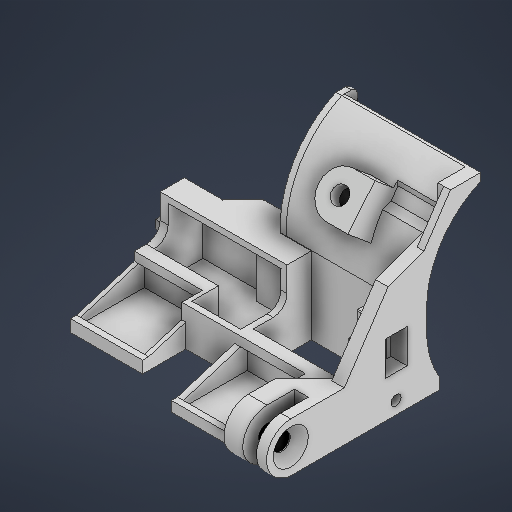
# Autodesk Inventor part: body-main2
Saved by Autodesk Inventor 2025 (Build 290162000, 162)
## iProperties
Created: 2025-03-21
Part Number: body-main2
Material: Všeobecné
Document SubType Name: Modeling
Designer: Simak
Density: 1 g/cm^3
Appearance: Výchozí
Author: Simak
Autodesk Inventor part; units mm, degrees
ref_plane "YZ Plane" through (0, 0, 0) normal (1, 0, 0) x (0, 1, 0)
ref_plane "XZ Plane" through (0, 0, 0) normal (0, 1, 0) x (-1, 0, 0)
ref_plane "XY Plane" through (0, 0, 0) normal (0, 0, 1) x (1, 0, 0)
sketch "Náčrt1" plane through (0, 0, 0) normal (1, 0, 0) x (0, 1, 0)
  circle A0 centre (13.5, 0) radius 16.5 construction
  circle A1 centre (15.5, 0) radius 16.5 construction
  circle A2 centre (11.5, 0) radius 16.5 construction
  line L0 (15.5, 16.5) -> (11.5, 16.5) construction
  line L1 (15.5, -16.5) -> (11.5, -16.5) construction
  circle A3 centre (5, 45.139) radius 5
  line L2 (0, 0) -> (0, 45.139)
  line L3 (10, 34.353) -> (22.965058, 25.70965)
  line L4 (10, 34.353) -> (10, 45.139)
  line L5 (22.965058, 25.70965) -> (27.5, 13.25)
  line L6 (27.5, 13.25) -> (33.5, 13.25)
  line L7 (33.5, 13.25) -> (25.577679, 18.531534)
  line L8 (33.5, 13.25) -> (33.5, 7.193747)
  line L9 (29, 13.25) -> (27.01942, 14.570383)
  arc A4 (13.5, -17.888544) -> (15.5, 18) centre (15.5, 0) ccw
  arc A5 (11.5, 18) -> (13.5, -17.888544) centre (11.5, 0) ccw
  line L10 (15.5, 18) -> (11.5, 18)
  line L11 (2.348497, 15.5) -> (0, 15.5)
  line L12 (33.5, 7.193747) -> (32, 7.193747)
  arc A6 (13.5, -19.497692) -> (15.5, 19.6) centre (15.5, 0) ccw
  arc A7 (11.5, 19.6) -> (13.5, -19.497692) centre (11.5, 0) ccw
  line L13 (11.5, 19.6) -> (15.5, 19.6)
  line L14 (21.6, 28.6) -> (0, 28.6) construction
  line L15 (0, 28.6) -> (0, 19.6)
  line L16 (0, 19.6) -> (21.6, 19.6)
  line L17 (21.6, 19.6) -> (21.6, 28.6) construction
  line L18 (35.6, 21.5) -> (34, 21.5) construction
  line L19 (34, 21.5) -> (34, -16) construction
  line L20 (34, -16) -> (35.6, -16) construction
  line L21 (35.6, -16) -> (35.6, 21.5) construction
  line L22 (35.6, 17.75) -> (34, 17.75) construction
  line L23 (33.21956, 14.55) -> (26.524235, 14.55) construction
  line L24 (10, 39.639) -> (0, 39.639)
  line L25 (10, 34.353) -> (9.85, 34.453)
  line L26 (9.85, 34.453) -> (9.85, 39.639)
  point P0 (26.391657, 16.295147)
  point P1 (33.5, 7.756288)
  point P2 (29.942905, 13.25)
  dimension "d0" = 33
  dimension "d1" = 2
  dimension "d2" = 2
  dimension "d3" = 13.5
  dimension "d4" = 10
  dimension "d5" = 45.139
  dimension "d6" = 10.786
  dimension "d8" = 123.69
  dimension "d10" = 13.25
  dimension "d11" = 33.5
  dimension "d12" = 6
  dimension "d16" = 1.5
  dimension "d17" = 36
  dimension "d18" = 36
  dimension "d20" = 1.5
  dimension "d21" = 1.6
  dimension "d23" = 9
  dimension "d24" = 21.6
  dimension "d25" = 0.5
  dimension "d26" = 1.6
  dimension "d27" = 37.5
  dimension "d28" = 3.75
  dimension "d29" = 20.5
  dimension "d30" = 3.2
  dimension "d41" = 5.5
  dimension "d45" = 9.85
  dimension "d86" = 70
  dimension "d103" = 15.5
  constraints: 54 end point, 17 point on circle, 11 point on line, 8 centre point, 8 perpendicular, 7 horizontal, 5 parallel, 5 tangent, 3 horizontal alignment, 3 vertical, 2 coincident, 2 collinear, 2 equal radius, 2 other
  measures "d0" diameter of A0
  measures "d1" distance of A0.centre A1.centre
  measures "d2" distance of A0.centre A2.centre
  measures "d3" distance of A0.centre L2.start
  measures "d4" diameter of A3
  measures "d5" vertical distance of A3.centre A0.centre
  measures "d6" vertical distance of A3.centre L3.start
  measures "d8" angle of L4 L3
  measures "d10" distance from line of A1.centre L6
  measures "d11" distance from line of L2 L6.end
  measures "d12" distance of L5.end L6.end
  measures "d16" distance of L5.end L9.start
  measures "d17" diameter of A4
  measures "d18" diameter of A5
  measures "d20" distance of L8.end L12.end
  measures "d21" radial gap between concentric circles of A4 A6
  measures "d23" distance of L16.end L14.start
  measures "d24" distance of L14.start L14.end
  measures "d25" distance between parallel lines of L20 L1
  measures "d26" distance of L19.end L20.end
  measures "d27" distance of L20.end L18.start
  measures "d28" distance between parallel lines of L18 L22
  measures "d29" distance from line of L19 A0.centre
  measures "d30" distance between parallel lines of L22 L23
  measures "d41" distance from line of A3.centre L24
  measures "d45" distance between parallel lines of L2 L26
  measures "d86" angle of L6 L5
  measures "d103" distance from line of A0.centre L11
extrude "Vysunutí1" add sketch "Náčrt1" against normal blind 2.5 contours L24 L26 L25 L3 L5 A6 L13 L16 L2 | L16 A7 L2 | A7 L13 A6 L5 A4 L10 A5 L11 L2 | L8 A6 L6 | L9 L6 A4 L5 | A6 L8 L12 A4 L6
extrude "Vysunutí3" add sketch "Náčrt1" against normal blind 49.5 contours L16 A7 L2 | A7 L13 A6 L5 A4 L10 A5 L11 L2 | A6 L6 L9 L5 | L9 L6 A4 L5 | A6 L8 L12 A4 L6
extrude "Vysunutí4" cut sketch "Náčrt1" against normal blind 10.5 contours A6 L6 L9 L5
extrude "Vysunutí5" add sketch "Náčrt1" against normal blind 1.35 contours L7 L6 A6 L5 | A6 L6 L9 L5
sketch "Náčrt2" plane through (0, 0, 0) normal (1, 0, 0) x (0, 0, -1)
  circle A0 centre (-45.139, 5) radius 4.85
  line L0 (-46.797798, 0.442491) -> (-45.582064, 0)
  line L1 (-19.6, 0) -> (-39.639, 0)
  line L2 (-39.639, 0) -> (-45.582064, 0)
  line L3 (-39.639, 9.85) -> (-39.639, 0)
  line L4 (-39.639, 9.85) -> (-45.139, 9.85)
  line L5 (-45.139, 8.889087) -> (-49.028087, 5)
  line L6 (-49.028087, 5) -> (-45.139, 1.110913)
  line L7 (-45.139, 1.110913) -> (-41.249913, 5)
  line L8 (-41.249913, 5) -> (-45.139, 8.889087)
  line L9 (-45.139, 8.889087) -> (-45.139, 5) construction
  line L10 (-45.139, 5) -> (-41.249913, 5) construction
  line L11 (-45.139, 5) -> (-45.139, 1.110913) construction
  point P0 (0, 0)
  dimension "d42" = 9.7
  dimension "d44" = 20
  dimension "d47" = 5.5
  constraints: 20 end point, 5 equal length, 4 perpendicular, 2 point on circle, 2 tangent, 1 centre point, 1 coincident, 1 collinear, 1 vertical
  measures "d42" diameter of A0
  measures "d44" angle of L2 L0
  measures "d47" distance of L7.end L5.start
extrude "Vysunutí6" add sketch "Náčrt2" against normal blind 8.5 contours A0 | A0 L4 L3 L2 L0 | L8 L7 L6 L5
sketch "Náčrt3" plane through (0, 0, 0) normal (1, 0, 0) x (0, 0, -1)
  arc A0 (-45.139, 9.85) -> (-46.797798, 0.442491) centre (-45.139, 5) ccw construction
  point P0 (0, 0)
  constraints: 1 coincident
hole "Díra1" at (0, 5, 45.139) direction (-1, 0, 0) diameter 3.4 end through all countersink diameter 7 countersink angle 90
sketch "Náčrt4" plane through (-8.5, 0, 0) normal (-1, 0, 0) x (0, 0, 1)
  line L0 (45.139, 1.110913) -> (41.249913, 5)
  line L1 (41.249913, 5) -> (45.139, 8.889087)
  line L2 (45.139, 8.889087) -> (49.028087, 5)
  line L3 (49.028087, 5) -> (45.139, 1.110913)
  point P0 (0, 0)
extrude "Vysunutí7" cut sketch "Náčrt4" against normal blind 2
sketch "Náčrt5" plane through (-2.5, 9.85, 34.453) normal (0, 1, 0) x (1, 0, 0)
  line L0 (2.5, -15.536) -> (-6, -15.536)
  line L1 (0.5, -15.536) -> (0.5, -5.186)
  line L2 (0.7, -12.386) -> (0.7, -8.986)
  line L3 (0.5, -5.186) -> (-2.25, -5.186)
  line L4 (-2.25, -5.186) -> (-2.25, -15.536)
  line L5 (2.5, 0) -> (2.5, -10.686)
  line L6 (2.5, -10.686) -> (-6, -10.686)
  line L7 (-6, -10.686) -> (-6, -5.186)
  line L8 (-6, -5.186) -> (0, 0.814)
  line L9 (0, 0) -> (0, 8.74335)
  line L10 (0, -5.186) -> (-6, -5.186)
  line L11 (0, -5.186) -> (0, 0)
  point P0 (2.5, 34.453)
  dimension "d59" = 2
  dimension "d60" = 2.75
  dimension "d61" = 5.5
  dimension "d62" = 45
  constraints: 8 end point, 2 perpendicular, 2 point on line, 1 parallel
  measures "d59" distance between parallel lines of L5 L1
  measures "d60" distance of L1.end L3.end
  measures "d61" distance between parallel lines of L3 L6
  measures "d62" angle of L10 L8
extrude "Vysunutí8" add sketch "Náčrt5" against normal up to surface (9.85 mm away) contours L10 L8 L9 L11 L3
extrude "Vysunutí9" cut sketch "Náčrt5" against normal through all contours L0 L4 L6 L1 | L6 L4 L3 L1
sketch "Náčrt6" plane through (-2.5, 0, 0) normal (-1, 0, 0) x (0, 0, 1)
  line L0 (19.6, 21.6) -> (28.6, 21.6)
  line L1 (28.6, 21.6) -> (28.6, 0)
  line L2 (19.6, 0) -> (19.6, 21.6)
  line L3 (19.6, 0) -> (33.639, 0)
  circle A0 centre (24.1, 2.54) radius 1
  line L4 (22.9, 13.2) -> (25.3, 13.2)
  line L5 (25.3, 13.2) -> (25.3, 8.4)
  line L6 (25.3, 8.4) -> (22.9, 8.4)
  line L7 (22.9, 8.4) -> (22.9, 13.2)
  line L8 (21.9, 14.2) -> (26.3, 14.2)
  line L9 (26.3, 14.2) -> (26.3, 7.4)
  line L10 (26.3, 7.4) -> (21.9, 7.4)
  line L11 (21.9, 7.4) -> (21.9, 14.2)
  line L12 (34.453, 9.85) -> (25.70965, 22.965058)
  line L13 (19.6, 18.85) -> (28.6, 18.85)
  arc A1 (13.25, 29.942905) -> (7.756288, 33.5) centre (0, 15.5) ccw
  arc A2 (19.6, 15.5) -> (7.756288, 33.5) centre (0, 15.5) ccw
  arc A3 (19.6, 15.5) -> (16.295147, 26.391657) centre (0, 15.5) ccw
  arc A4 (16.295147, 26.391657) -> (13.25, 29.942905) centre (0, 15.5) ccw
  line L14 (19.6, 18.85) -> (19.31159, 18.85)
  point P0 (0, 0)
  point P1 (24.1, 21.6)
  point P2 (24.1, 13.2)
  point P3 (28.453015, 18.85)
  point P4 (28.6, 18.629522)
  dimension "d67" = 2.54
  dimension "d68" = 2
  dimension "d69" = 2.4
  dimension "d70" = 4.8
  dimension "d71" = 8.4
  dimension "d72" = 1
  dimension "d77" = 2.75
  constraints: 20 end point, 4 parallel, 3 horizontal, 2 midpoint, 2 perpendicular, 2 point on line, 2 vertical alignment, 1 centre point, 1 point on circle, 3 other
  measures "d67" distance from line of L3 A0.centre
  measures "d68" diameter of A0
  measures "d69" distance of L4.start L4.end
  measures "d70" distance of L4.end L5.end
  measures "d71" distance between parallel lines of L3 L6
  measures "d72" distance between parallel lines of L7 L11
  measures "d77" distance between parallel lines of L0 L13
extrude "Vysunutí10" add sketch "Náčrt6" along normal blind 2.5 contours L13 L12 L1 L3 L2 | L2 A2 L14
extrude "Vysunutí11" cut sketch "Náčrt6" against normal through all contours A0 | L4 L5 L6 L7 | L8 L9 L10 L11
sketch "Náčrt7" plane through (-5, 0, 0) normal (-1, 0, 0) x (0, 0, 1)
  line L0 (19.6, 0) -> (19.6, 15.5)
  line L1 (19.6, 3.25) -> (28.6, 3.25)
  line L2 (28.6, 0) -> (28.6, 18.629522)
  line L3 (28.6, 5.5) -> (27.1, 5.5)
  line L4 (27.1, 5.5) -> (27.1, 13)
  line L5 (27.1, 13) -> (28.6, 13)
  line L6 (19.6, 13) -> (21.1, 13)
  line L7 (21.1, 13) -> (21.1, 5.5)
  line L8 (21.1, 5.5) -> (19.6, 5.5)
  circle A0 centre (24.1, 2.54) radius 1
  line L9 (19.6, 0) -> (28.6, 0)
  circle A1 centre (24.1, 2.54) radius 2
  line L10 (19.6, 0) -> (19.6, 15.5)
  line L11 (19.6, 0) -> (28.6, 0)
  line L12 (28.6, 0) -> (28.6, 18.629522)
  line L13 (28.453015, 18.85) -> (19.31159, 18.85)
  line L14 (21.9, 14.2) -> (26.3, 14.2)
  line L15 (26.3, 14.2) -> (26.3, 7.4)
  line L16 (26.3, 7.4) -> (21.9, 7.4)
  line L17 (21.9, 7.4) -> (21.9, 14.2)
  circle A2 centre (24.1, 2.54) radius 1
  line L18 (28.6, 18.629522) -> (28.453015, 18.85)
  arc A3 (19.6, 15.5) -> (19.31159, 18.85) centre (0, 15.5) ccw
  point P0 (0, 0)
  point P1 (28.6, 18.85)
  point P2 (28.6, 18.85)
  point P3 (22.230267, 3.25)
  point P4 (25.969733, 3.25)
  dimension "d78" = 1.5
  dimension "d79" = 7.5
  dimension "d80" = 13
  dimension "d82" = 3.25
  dimension "d83" = 1
  constraints: 14 end point, 8 point on line, 4 perpendicular, 2 equal length, 2 horizontal, 1 centre point, 1 horizontal alignment
  measures "d78" distance of L4.end L5.end
  measures "d79" distance of L6.end L7.end
  measures "d80" distance between parallel lines of L9 L6
  measures "d82" distance between parallel lines of L9 L1
  measures "d83" radial gap between concentric circles of A0 A1
extrude "Vysunutí12" cut sketch "Náčrt7" against normal blind 1.75 contours L0 L8 L7 L6 A3 L13 L18 L2 L5 L4 L3 L1 A1 | A0 L1 | L1 A0
sketch "Náčrt8" plane through (0, 32, 7.193747) normal (0, 0, -1) x (-1, 0, 0)
  line L0 (0, 1.5) -> (49.5, 1.5)
  line L1 (49.5, -32) -> (49.5, -16.5)
  line L2 (49.5, -16.5) -> (49.5, 1.5)
  line L3 (49.5, 1.5) -> (49.5, 0)
  line L4 (49.5, 0) -> (49.5, -16.5)
  line L5 (49.5, -16.5) -> (49.5, -20.5)
  line L6 (49.5, -20.5) -> (49.5, -29.651503)
  line L7 (49.5, -29.651503) -> (49.5, -32)
  line L8 (0, -32) -> (49.5, -32)
  line L9 (0, -24.6) -> (0, -17.8)
  line L10 (0, -17.8) -> (0, -24.6)
  line L11 (0, -30.5) -> (0, -23.5)
  line L12 (0, 1.5) -> (0, -6.422321)
  line L13 (0, -6.422321) -> (0, -9.034942)
  line L14 (0, -9.034942) -> (0, -22.15)
  line L15 (0, -22.15) -> (0, -31.557509)
  line L16 (0, -31.557509) -> (0, -32)
  line L17 (0, -32) -> (0, -29.651503)
  line L18 (0, -29.651503) -> (0, -20.5)
  line L19 (0, -20.5) -> (0, -16.5)
  line L20 (0, -16.5) -> (0, 0)
  line L21 (0, 0) -> (0, 1.5)
  line L22 (0, -32) -> (0, -35) construction
  line L23 (0, -35) -> (25, -35) construction
  line L24 (25, -35) -> (25, -2) construction
  line L25 (25, -2) -> (0, -2) construction
  line L26 (1.111468, 0) -> (26.090605, -1.021144)
  line L27 (26.090605, -1.021144) -> (24.742695, -33.993604)
  line L28 (24.742695, -33.993604) -> (-0.236442, -32.97246)
  line L29 (-0.236442, -32.97246) -> (1.111468, 0)
  line L30 (24.742695, -33.993604) -> (49.5, -28.2) construction
  line L31 (49.5, -28.2) -> (25.41665, -17.507374) construction
  line L32 (25, -18.5) -> (49.5, -28.2) construction
  line L33 (25, -35) -> (49.5, -28.2) construction
  line L34 (0.316161, -37) -> (-1.020895, -4.027098)
  line L35 (-1.020895, -4.027098) -> (23.958577, -3.014177)
  line L36 (23.958577, -3.014177) -> (25.295633, -35.987079)
  line L37 (25.295633, -35.987079) -> (0.316161, -37)
  line L38 (24.627105, -19.500628) -> (49.5, -28.2) construction
  line L39 (25.295633, -35.987079) -> (49.5, -28.2) construction
  circle A0 centre (49.5, -28.2) radius 3.8
  line L40 (49.5, -23.6) -> (25.5, -23.6)
  line L41 (25.5, -23.6) -> (25.5, -18.5)
  line L42 (35, -18.5) -> (40.1, -23.6)
  line L43 (25.5, -18.5) -> (35, -18.5)
  line L44 (27.194504, 1.5) -> (26, -27.719862)
  line L45 (26, -32) -> (26, -27.719862)
  point P0 (0, -30.46)
  point P1 (0, -28.46)
  point P2 (26.376907, -18.5)
  dimension "d87" = 33
  dimension "d88" = 25
  dimension "d89" = 13.5
  dimension "d90" = 3.8
  dimension "d91" = 2
  dimension "d92" = 2
  dimension "d94" = 8.4
  dimension "d95" = 24
  dimension "d96" = 9.5
  dimension "d97" = 13.5
  dimension "d98" = 45
  dimension "d99" = 1
  dimension "d104" = 1
  dimension "d144" = 2.32208
  constraints: 48 end point, 10 perpendicular, 8 equal length, 8 point on line, 3 midpoint, 3 vertical, 1 coincident, 1 horizontal, 1 parallel, 1 vertical alignment, 2 other
  measures "d87" distance of L23.end L24.end
  measures "d88" distance of L24.end L25.end
  measures "d89" distance from line of L8 L32.start
  measures "d90" distance from line of L8 L30.end
  measures "d91" distance from line of L25 L26.start
  measures "d92" distance from line of L34.start L23
  measures "d94" distance between parallel lines of L8 L40
  measures "d95" distance of L40.start L40.end
  measures "d96" distance of L41.end L43.end
  measures "d97" distance between parallel lines of L8 L43
  measures "d98" angle of L40 L42
  measures "d99" distance between parallel lines of L27 L44
  measures "d104" distance between parallel lines of L24 L45
  measures "d144" angle of L39 L33
extrude "Vysunutí13" cut sketch "Náčrt8" against normal through all contours L0 L2 L1 L40 L42 L43 L44
sketch "Náčrt10" plane through (0, 0, 15.5) normal (0, 0, -1) x (-1, 0, 0)
  line L0 (49.5, 8.4) -> (25.5, 8.4)
  line L1 (49.5, 11.5) -> (49.5, 2.348497)
  line L2 (49.5, 8.4) -> (49.5, 2.348497)
  line L3 (49.5, 2.348497) -> (49.5, 0)
  line L4 (49.5, 0) -> (49.5, 8.4)
  line L5 (0, 0) -> (49.5, 0)
  line L6 (35, 13.5) -> (40.1, 8.4)
  line L7 (25.5, 13.5) -> (35, 13.5)
  line L8 (27.194504, 33.5) -> (26, 4.280138)
  line L9 (26, 0) -> (26, 4.280138)
  point P0 (26.376907, 13.5)
  point P1 (49.5, 3.8)
  constraints: 1 other
extrude "Vysunutí14" add sketch "Náčrt10" against normal up to next
sketch "Náčrt11" plane through (0, 0, 15.5) normal (0, 0, -1) x (-1, 0, 0)
  circle A0 centre (49.5, 3.8) radius 8.417268
  circle A1 centre (49.5, 3.8) radius 15
  line L0 (41.082732, 3.8) -> (34.5, 3.8)
  line L1 (41.082732, 3.8) -> (49.5, 3.8) construction
  line L2 (0, 0) -> (49.5, 0)
  line L3 (26, 4.280138) -> (26, 2.348497)
  line L4 (41.089644, 3.458959) -> (34.512317, 3.192247)
  circle A2 centre (49.5, 3.8) radius 8.917268
  circle A3 centre (49.5, 3.8) radius 14.5
  point P0 (35.011907, 3.212506)
  point P1 (35.506787, 0)
  point P2 (38.817748, 0)
  point P3 (40.590054, 3.4387)
  point P4 (35.506787, 0)
  point P5 (41.432927, 0)
  point P6 (41.989314, 0)
  point P7 (34.989314, 0)
  dimension "d146" = 2.32208
  dimension "d147" = 0.5
  dimension "d148" = 0.5
  dimension "d149" = 15
  dimension "d151" = 7
  constraints: 6 end point, 6 point on circle, 5 point on line, 2 centre point, 2 coincident, 1 collinear, 1 horizontal, 6 other
  measures "d146" angle of L0 L4
  measures "d149" distance of L0.end A0.centre
  measures "d151" distance of point (41.989, 0) point (34.989, 0)
extrude "Vysunutí15" add sketch "Náčrt11" along normal blind 5 contours L2 A3 L4 A2
sketch "Náčrt12" plane through (-27.194504, 33.5, 7.193747) normal (-0.9991655, -0.0408458, 0) x (0, 0, 1)
  line L0 (12.406253, -18.015034) -> (12.406253, -20.016705)
  ellipse E0 centre (-7.193747, -18.015034) end of major axis (-7.193747, -37.631405) minor radius 19.6 (12.406253, -18.015034) -> (0.56254, 0) ccw
  line L1 (0, 0) -> (0.56254, 0)
  line L2 (0, -1.501253) -> (0, 0)
  ellipse E1 centre (-7.193747, -18.015034) end of major axis (-7.193747, 0) minor radius 18 (10.806253, -18.015034) -> (0, -1.501253) ccw
  line L3 (10.806253, -20.016705) -> (10.806253, -18.015034)
  line L4 (10.806253, -20.016705) -> (12.406253, -20.016705)
  line L5 (-2.5, -3.228477) -> (-2.5, 2.5)
  line L6 (-2.5, 2.5) -> (1.062535, 2.5)
  line L7 (14.906253, -18.015034) -> (14.906253, -22.516705)
  line L8 (14.906253, -22.516705) -> (8.306253, -22.516705)
  line L9 (8.306253, -22.516705) -> (8.306253, -18.015034)
  line L10 (0, 0) -> (-2.5, 0)
  circle A0 centre (1.25, -3.75) radius 3.75
  line L11 (8.306253, -20.016705) -> (10.806253, -20.016705)
  line L12 (10.806253, -20.016705) -> (12.406253, -20.016705)
  line L13 (-0.625, -6.997595) -> (6.76093, -11.261864)
  circle A1 centre (-1.40165, -1.09835) radius 1.09835
  line L14 (-2.5, -3.228477) -> (-2.5, -3.75)
  line L15 (8.306253, -18.015034) -> (8.306253, -12.154056)
  line L16 (8.306253, -12.154056) -> (6.76093, -11.261864)
  spline S0 degree 5 poles (1.062536, 2.500002) (3.547609, 1.498411) (5.880817, 0.120039) (7.98602, -1.604347) (11.536372, -5.556933) (13.783796, -10.366122) (14.532109, -12.867419) (14.906261, -15.441226) (14.906256, -18.015034) knots 0 0 0 0 0 0 0.51004293 0.51004293 0.51004293 1 1 1 1 1 1
  spline S1 degree 5 poles (8.306175, -18.015034) (8.306516, -14.096819) (7.071568, -10.178394) (4.594456, -6.782604) (1.233576, -4.416213) (-2.50004, -3.228604) knots 0 0 0 0 0 0 1 1 1 1 1 1
  point P0 (-7.193747, -34.582823)
  point P1 (8.306253, -19.664488)
  point P2 (-1.40165, 0)
  point P3 (-2.5, -1.09835)
  dimension "d113" = 60
  dimension "d114" = 7.5
  constraints: 20 end point, 5 tangent, 3 parallel, 3 point on circle, 2 centre point, 2 point on line, 2 vertical, 1 collinear, 1 perpendicular, 12 other
  measures "d113" angle of L13 L3
  measures "d114" diameter of A0
extrude "Vysunutí16" add sketch "Náčrt12" along normal blind 1.2 contours L0 L4 L3 E1 A0 E0 | A0 E1 L2 E0 | L11 L9 L15 L16 S1 A0 E1 L3 | A0 L2 L1 E0 | A0 A1 L10 L2 | L2 E1 A0 S1 A1 | A1 A0 | A0 A1 | S1 L13 A0 | A0 S1 | A0 S1 L5 A1 | A0 L14 S1
sketch "Náčrt13" plane through (0, 0, 15.5) normal (0, 0, -1) x (-1, 0, 0)
  line L0 (49.5, 0) -> (49.5, 8.4)
  circle A0 centre (49.5, 3.8) radius 1.5
  line L1 (49.5, 0.682309) -> (46.8, 2.241154)
  line L2 (46.8, 2.241154) -> (46.8, 5.358846)
  line L3 (46.8, 5.358846) -> (49.5, 6.917691)
  line L4 (49.5, 6.917691) -> (52.2, 5.358846)
  line L5 (52.2, 5.358846) -> (52.2, 2.241154)
  line L6 (52.2, 2.241154) -> (49.5, 0.682309)
  line L7 (41.432927, 0) -> (49.5, 0)
  line L8 (49.5, 8.4) -> (40.1, 8.4)
  line L9 (46.8, 5.358846) -> (46.8, 8.4)
  point P0 (0, 0)
  point P1 (39.35, 0)
  point P2 (49.5, 2.3)
  point P3 (49.5, 5.3)
  dimension "d117" = 5.4
  dimension "d118" = 3.8
  dimension "d119" = 3
  constraints: 14 end point, 3 point on line, 1 centre point, 1 coincident, 1 perpendicular, 13 other
  measures "d117" distance between parallel lines of L2 L5
  measures "d118" distance from line of L7 point (49.5, 3.8)
  measures "d119" diameter of A0
extrude "Vysunutí17" cut sketch "Náčrt13" against normal up to next
extrude "Vysunutí18" add sketch "Náčrt13" against normal blind 1 contours L3 L9 L8 L0 | L0 A0 L1 L2 L3
ref_plane "Pracovní rovina1" through (0, 0, 18.9) normal (0, 0, -1) x (-1, 0, 0)
sketch "Náčrt14" plane through (0, 0, 18.9) normal (0, 0, -1) x (-1, 0, 0)
  line L0 (46.8, 5.358846) -> (49.5, 6.917691)
  line L1 (46.8, 2.241154) -> (46.8, 5.358846)
  line L2 (49.5, 0.682309) -> (46.8, 2.241154)
  arc A0 (49.5, 5.3) -> (49.5, 2.3) centre (49.5, 3.8) ccw
  line L3 (49.5, 0) -> (49.5, 8.4)
  line L4 (40.1, 8.4) -> (46.8, 8.4)
  line L5 (49.5, 8.4) -> (46.8, 8.4)
  line L6 (46.8, 8.4) -> (46.8, 2.241154)
  line L7 (46.8, 8.4) -> (49.5, 8.4)
  circle A1 centre (49.5, 3.8) radius 4.6
  line L8 (44.9, 3.8) -> (44.9, 0)
  line L9 (41.432927, 0) -> (49.5, 0)
  line L10 (46.8, 2.241154) -> (46.8, 0)
  point P0 (0, 0)
  point P1 (39.35, 0)
  point P2 (46.8, 0.075755)
  point P3 (46.907704, 0)
  point P4 (46.8, 7.524245)
  constraints: 6 end point, 2 point on circle, 2 point on line, 1 centre point, 1 coincident, 1 horizontal, 1 perpendicular, 1 tangent, 1 vertical
extrude "Vysunutí19" add sketch "Náčrt14" against normal blind 1 contours L0 L3 A0 L2 L1
extrude "Vysunutí20" add sketch "Náčrt14" against normal blind 3.8 contours L6 A1 L3 L0 | L1 L10 A1 L6 | L2 L3 L9 A1 L10 | L6 L5 A1 | L10 L9 L8 A1 | A1 L9 L10
extrude "Vysunutí21" add sketch "Náčrt14" against normal blind 5.8 contours L2 L3 L9 A1 L10 | A1 L9 L10
sketch "Náčrt16" plane through (0, 0, 15.5) normal (0, -1, 0) x (1, 0, 0)
  line L0 (-46.8, 7.2) -> (-46.8, 9.2) projected
  line L1 (-46.8, 9.2) -> (-41.955, 4.1)
  line L2 (-5, 4.1) -> (-44.9, 4.1) projected
  line L3 (-46.8, 7.2) -> (-44.9, 7.2) projected
  line L4 (-44.9, 4.1) -> (-44.9, 7.2) projected
  line L5 (-46.8, 4.4) -> (-46.8, 7.2) projected
  line L6 (-46.8, 4.4) -> (-46.8, 7.2) projected
  line L7 (-46.8, 4.1) -> (-44.9, 4.1) projected
  line L8 (-49.5, 4.4) -> (-46.8, 4.4) projected
  line L9 (-46.8, 4.4) -> (-46.8, 4.1)
  point P0 (0, -15.5)
  point P1 (-46.8, 7.2)
  point P2 (-3.25, 3.85)
  constraints: 4 end point, 1 perpendicular, 1 point on line, 2 other
extrude "Vysunutí22" add sketch "Náčrt16" against normal up to surface contours L0 L1 L3 surface through (-46.8, 2.241154, 18.9) normal (-0.5, 0.8660254, 0)
sketch "Náčrt25" plane through (-5, 3.25, 19.6) normal (0, 0, 1) x (1, 0, 0)
  arc A0 (-39.9, 0.55) -> (-41.8, 4.274245) centre (-44.5, 0.55) ccw
  line L0 (-39.9, 0.55) -> (-39.9, -3.25)
  line L1 (0, -3.25) -> (-39.9, -3.25)
  line L2 (0, -3.25) -> (0, 0)
  line L3 (0, 0) -> (1.75, 0)
  line L4 (1.75, 0) -> (1.75, 2.25)
  line L5 (0, 2.25) -> (1.75, 2.25)
  line L6 (0, 2.25) -> (0, 9.75)
  line L7 (0, 9.75) -> (1.75, 9.75)
  line L8 (1.75, 9.75) -> (1.75, 12.25)
  line L9 (1.75, 12.25) -> (-21.458667, 12.25)
  line L10 (-21.458667, 12.25) -> (-22.657665, 12.200985)
  line L11 (-22.577909, 10.25) -> (-22.657665, 12.200985)
  line L12 (-22.577909, 10.25) -> (-30, 10.25)
  line L13 (-30, 10.25) -> (-35.1, 5.15)
  line L14 (-35.1, 5.15) -> (-41.8, 5.15)
  line L15 (-41.8, 5.15) -> (-41.8, 4.274245)
  line L16 (-40.2, -1.65) -> (-15.2, -1.65)
  line L17 (-15.2, -1.65) -> (-15.2, 11.35)
  line L18 (-13.6, 12.95) -> (-13.6, -3.25)
  arc A1 (-39.9, 0.55) -> (-44.5, 5.15) centre (-44.5, 0.55) ccw
  line L19 (-40.2, -1.65) -> (-40.2, 11.35)
  line L20 (-13.6, 12.95) -> (-41.8, 12.95)
  line L21 (-40.2, 11.35) -> (-15.2, 11.35)
  line L22 (-41.8, 12.95) -> (-41.8, 4.274245)
  line L23 (-41.8, 4.274245) -> (-41.8, -3.25)
  line L24 (-36.432927, -3.25) -> (-44.5, -3.25)
  line L25 (-41.8, -1.008846) -> (-41.8, 2.108846)
  line L26 (-41.8, 2.108846) -> (-41.8, -1.008846)
  line L27 (-40.2, -1.65) -> (-40.2, -3.25)
  point P0 (5, -3.25)
  point P1 (-40.2, 2.184013)
  point P2 (-39.9, -1.65)
  point P3 (-41.8, 4.274245)
  dimension "d237" = 1.6
  dimension "d238" = 25
  dimension "d240" = 13
  dimension "d241" = 1.6
  dimension "d242" = 1.6
  dimension "d243" = 1.6
  constraints: 19 end point, 4 perpendicular, 4 point on line, 3 horizontal, 2 vertical, 1 point on circle
  measures "d237" distance between parallel lines of L1 L16
  measures "d238" distance between parallel lines of L19 L17
  measures "d240" distance of L16.end L17.end
  measures "d241" distance between parallel lines of L17 L18
  measures "d242" distance between parallel lines of L20 L21
  measures "d243" distance between parallel lines of L22 L19
extrude "Vysunutí34" cut sketch "Náčrt25" along normal up to next contours L0 L16 L19 A0 | L0 L24 L27 L16
sketch "Náčrt30" plane through (-45.2, 0, 19.6) normal (1, 0, 0) x (0, 0, -1)
  line L0 (-3.1, 3.164915) -> (-3.1, 5.434013)
  line L1 (-3.415789, 3.164915) -> (-3.1, 3.164915)
  line L2 (-3.415789, 0) -> (-3.415789, 3.164915)
  line L3 (0, 0) -> (-3.415789, 0)
  line L4 (0, 5.434013) -> (0, 0)
  line L5 (-3.1, 5.434013) -> (0, 5.434013)
  line L6 (-3.1, 5.434013) -> (0, 5.434013)
  line L7 (0, 7.524245) -> (0, 5.434013)
  line L8 (-3.1, 5.434013) -> (-3.1, 7.524245)
  line L9 (-3.415789, 0) -> (-3.415789, 3.164915)
  line L10 (-3.415789, 3.164915) -> (-5.1, 2.241154)
  line L11 (-5.1, 0) -> (-5.1, 2.241154)
  line L12 (-3.415789, 0) -> (-5.1, 0)
  line L13 (0, 13.5) -> (0, 8.4)
  line L14 (4.1, 13.5) -> (0, 13.5)
  line L15 (4.1, 8.4) -> (4.1, 13.5)
  line L16 (4.1, 8.4) -> (0, 8.4)
  line L17 (0, 13.5) -> (4.1, 13.5)
  line L18 (0, 13.5) -> (0, 15.450985)
  arc A0 (11.843712, 33.450985) -> (0, 15.450985) centre (19.6, 15.450985) ccw
  line L19 (11.843712, 33.450985) -> (13.807903, 33.450985)
  ellipse E0 centre (13.807903, 32.353552) end of major axis (12.709554, 32.353552) minor radius 1.097433 (14.906253, 32.353552) -> (13.807903, 33.450985) ccw
  line L20 (14.906253, 32.353552) -> (14.906253, 29.704115)
  ellipse E1 centre (11.156253, 29.704115) end of major axis (7.406253, 29.704115) minor radius 3.74687 (13.031253, 26.45923) -> (14.906253, 29.704115) ccw
  line L21 (13.031253, 26.45923) -> (4.1, 21.307072)
  line L22 (4.1, 21.307072) -> (4.1, 13.5)
  line L23 (2.1, 14.2) -> (2.1, 1.2)
  line L24 (2.1, 1.2) -> (-7.6, 1.2)
  line L25 (-7.6, 1.2) -> (-7.6, 14.2)
  line L26 (-7.6, 14.2) -> (2.1, 14.2)
  line L27 (-8.8, 15.4) -> (-8.8, 0)
  line L28 (-8.8, 0) -> (3.3, 0)
  line L29 (3.3, 0) -> (3.3, 15.4)
  line L30 (3.3, 15.4) -> (-8.8, 15.4)
  line L31 (-7.6, 1.2) -> (-12.9, 1.2) construction
  line L32 (-12.9, 1.2) -> (-12.9, 14.2) construction
  line L33 (-12.9, 14.2) -> (-7.6, 14.2) construction
  arc A1 (12.406253, 32) -> (1.6, 15.5) centre (19.6, 15.5) ccw
  arc A2 (12.406253, 32) -> (1.6, 15.5) centre (19.6, 15.5) ccw
  line L34 (1.6, 11.5) -> (1.6, 15.5)
  line L35 (1.6, 11.5) -> (1.6, 15.5)
  line L36 (-4.85, 15.4) -> (-4.85, 14.2)
  line L37 (-4.85, 14.2) -> (-4.85, 10.45)
  arc A3 (-7.6, 7.7) -> (-4.85, 10.45) centre (-7.6, 10.45) ccw
  line L38 (0, 14.2) -> (0, 1.2) construction
  line L39 (-7.6, 7.7) -> (-8.8, 7.7)
  circle A4 centre (2.1, 10.5) radius 2.1
  line L40 (0, 7.524245) -> (-3.1, 7.524245)
  point P0 (19.6, 0)
  point P1 (0, 10.5)
  point P2 (0, 15.4)
  point P3 (3.3, 8.4)
  point P4 (2.1, 8.4)
extrude "Vysunutí38" cut sketch "Náčrt30" along normal blind 12.8 contours L1 L10 L11 L24 L25 A3 L37 L26 L18 L13 L16 L23 L4 L7 L40 L8 L0 | L0 L5 L4 L24 L2 L1 | L8 L40 L7 L5 | L2 L24 L11 L10 | A4 L23 | L16 L13 A4 | L25 L26 L37 A3 | A4 L34 L14 L23 | L13 L14 L34 A4 | L14 L34 L26 L23 | L18 L26 L34 L14
extrude "Vysunutí39" add sketch "Náčrt30" against normal up to surface (1.6 mm away) contours L1 L10 L11 L24 L25 A3 L37 L26 L18 L13 L16 L23 L4 L7 L40 L8 L0 | L0 L5 L4 L24 L2 L1 | L8 L40 L7 L5 | L2 L24 L11 L10 | L24 L4 L3 L2 | L2 L12 L11 L24 | L24 L23 L16 L29 L28 L4 | L11 L28 L27 L39 L25 L24 | L16 L13 A4 | L36 L30 L18 L26
extrude "Vysunutí40" add sketch "Náčrt30" along normal up to surface (12.8 mm away) contours L24 L4 L3 L2 | L2 L12 L11 L24 | L11 L28 L27 L39 L25 L24 | L36 L30 L18 L26
sketch "Náčrt31" plane through (-45.2, 10.5, 19.6) normal (0, 0, -1) x (-1, 0, 0)
  line L0 (1.6, 0) -> (1.6, 4.9)
  line L1 (1.6, 4.9) -> (-12.8, 4.9)
  line L2 (-12.8, 4.9) -> (-12.8, 3.7)
  line L3 (0, 3.7) -> (-12.8, 3.7)
  line L4 (0, 0) -> (0, 3.7)
  line L5 (0, 0) -> (1.6, 0)
  line L6 (-5.1, -2.1) -> (-10.2, 3)
  line L7 (-10.2, 3) -> (-12.1, 4.9)
  line L8 (-12.8, 4.9) -> (-17.544419, 4.9)
  line L9 (-17.302939, 10.807072) -> (-17.622091, 3)
  line L10 (-10.2, 3) -> (-17.622091, 3)
  line L11 (-10.2, 3) -> (-10.2, 4.9)
  line L12 (-12.8, 3.7) -> (-12.8, 3)
  point P0 (-45.2, -10.5)
  point P1 (-10.2, 3.7)
  constraints: 8 end point, 4 point on line, 2 vertical, 1 collinear, 1 horizontal
extrude "Vysunutí41" add sketch "Náčrt31" along normal up to surface (4.1 mm away) contours L11 L3 L7 L1 | L7 L3 L2 L1 | L11 L7 L3 | L2 L12 L10 L9 L8 | L7 L10 L12 L3
extrude "Vysunutí42" cut sketch "Náčrt31" along normal up to surface (2.1 mm away) contours L11 L7 L3 | L7 L10 L12 L3
chamfer "Zkosení8" distance 4.1 angle 45 1 edges at (-35, 14.8, 19.6)
sketch "Náčrt32" plane through (-32.4, 0, 19.6) normal (-1, 0, 0) x (0, 0, 1)
  line L0 (12.9, 14.2) -> (7.6, 14.2) projected
  line L1 (12.9, 1.2) -> (12.9, 14.2) projected
  line L2 (7.6, 1.2) -> (12.9, 1.2) projected
  line L3 (0, 14.2) -> (0, 1.2) projected
  line L4 (7.6, 14.2) -> (0, 14.2)
  line L5 (0, 1.2) -> (7.6, 1.2)
  line L6 (14.1, 15.4) -> (14.1, 0)
  line L7 (14.1, 0) -> (-1.2, 0)
  line L8 (-1.2, 0) -> (-1.2, 15.4)
  line L9 (14.1, 15.4) -> (-1.2, 15.4)
  line L10 (0, 15.4) -> (-4.1, 15.4) projected
  line L11 (-4.1, 0) -> (5.1, 0) projected
  line L12 (4.85, 15.4) -> (4.85, 10.45) projected
  line L13 (4.85, 14.2) -> (4.85, 10.45) projected
  line L14 (4.85, 14.2) -> (4.85, 15.4) projected
  line L15 (12.9, 7.7) -> (14.1, 7.7)
  line L16 (7.6, 7.7) -> (8.8, 7.7) projected
  line L17 (8.8, 7.7) -> (7.6, 7.7) projected
  arc A0 (4.85, 10.45) -> (7.6, 7.7) centre (7.6, 10.45) ccw projected
  arc A1 (4.85, 10.45) -> (7.6, 7.7) centre (7.6, 10.45) ccw projected
  line L18 (8.8, 7.7) -> (8.8, 0) projected
  line L19 (8.8, 7.7) -> (12.9, 7.7)
  point P0 (-19.6, 0)
  dimension "d279" = 1.2
  dimension "d280" = 1.2
  constraints: 16 end point, 2 midpoint, 1 collinear, 1 horizontal, 1 parallel, 1 perpendicular, 1 point on line, 1 other
  measures "d279" distance between parallel lines of L6 L1
  measures "d280" distance between parallel lines of L0 L9
extrude "Vysunutí43" add sketch "Náčrt32" against normal blind 10.95 contours L15 L6 L7 L18 L2 L1 | L1 L2 L18 L19 | L12 A0 L16 L18 L2 L5 L3 L4 | L4 L3 L5 L2 L18 L7 L8 L9 L12
extrude "Vysunutí44" cut sketch "Náčrt32" against normal blind 9.75 contours L1 L2 L18 L19 | L12 A0 L16 L18 L2 L5 L3 L4
extrude "Vysunutí45" add sketch "Náčrt32" along normal blind 0.8 contours L15 L6 L7 L18 L2 L1 | L1 L2 L18 L19
sketch "Náčrt34" plane through (-33.2, 0, 19.6) normal (-1, 0, 0) x (0, 0, 1)
  line L0 (8.8, 0) -> (8.8, 7.7)
  line L1 (8.8, 0) -> (14.1, 0)
  line L2 (14.1, 0) -> (14.1, 7.7)
  line L3 (14.1, 7.7) -> (8.8, 7.7)
  line L4 (10, 7.7) -> (10, 5.95)
  line L5 (10, 5.95) -> (8.8, 5.95)
  line L6 (10, 5.95) -> (21.55, 2.4)
  line L7 (21.55, 2.4) -> (22.75, 2.4)
  line L8 (22.75, 2.4) -> (22.75, 0)
  line L9 (14.039, 0) -> (20.039, 0)
  line L10 (14.1, 0) -> (0, 0)
  line L11 (8.8, 0) -> (14.1, 0)
  line L12 (8.8, 0) -> (5.1, 0)
  line L13 (-4.1, 0) -> (5.1, 0)
  line L14 (-4.1, 0) -> (-9.1, 0)
  line L15 (-4.1, 0) -> (-9.1, 0)
  line L16 (25.982064, 0) -> (-4.1, 0)
  line L17 (25.982064, 0) -> (20.039, 0)
  line L18 (20.039, 0) -> (25.982064, 0)
  line L19 (20.039, 0) -> (25.982064, 0)
  line L20 (14.039, 0) -> (20.039, 0)
  line L21 (9, 0) -> (14.039, 0)
  line L22 (0, 0) -> (9, 0)
  line L23 (21.55, 2.4) -> (21.55, 0)
  line L24 (0, 1.2) -> (-2.1, 1.2)
  line L25 (7.6, 1.2) -> (-2.1, 1.2)
  line L26 (7.6, 1.2) -> (12.9, 1.2)
  line L27 (12.9, 1.2) -> (0, 1.2)
  line L28 (12.9, 1.2) -> (0, 1.2)
  line L29 (12.9, 1.2) -> (21.55, 1.2)
  point P0 (-19.6, 0)
  point P1 (8.8, 1.2)
  point P2 (22.75, 0)
  point P3 (14.1, 4.689827)
  dimension "d288" = 1.2
  dimension "d289" = 1.2
  dimension "d290" = 4.75
  dimension "d291" = 1.2
  dimension "d292" = 12.75
  constraints: 14 end point, 4 point on line, 3 perpendicular, 1 collinear, 1 midpoint, 1 vertical
  measures "d288" distance between parallel lines of L29 L7
  measures "d289" distance of L6.end L7.end
  measures "d290" distance between parallel lines of L26 L5
  measures "d291" distance of L4.end L5.end
  measures "d292" distance between parallel lines of L23 L0
extrude "Vysunutí46" add sketch "Náčrt34" along normal up to surface (13.6 mm away) contours L0 L3 L4 L5 | L26 L29 L2 L1 L0 | L29 L23 L16 L9 L2 | L7 L8 L16 L23
sketch "Náčrt35" plane through (-46.8, 2.241154, 16.5) normal (-1, 0, 0) x (0, 0, 1)
  line L0 (3.4, 0) -> (3.4, 3.117691)
  line L1 (3.4, 0) -> (8.2, 0)
  line L2 (8.2, -2.241154) -> (8.2, 0)
  line L3 (25.85, -2.241154) -> (8.2, -2.241154)
  line L4 (25.85, 0.158846) -> (25.85, -2.241154)
  line L5 (24.65, 0.158846) -> (25.85, 0.158846)
  line L6 (24.65, -1.041154) -> (24.65, 0.158846)
  line L7 (11.9, -1.041154) -> (24.65, -1.041154)
  line L8 (11.9, 3.708846) -> (11.9, -1.041154)
  line L9 (13.1, 3.708846) -> (11.9, 3.708846)
  line L10 (13.1, 5.458846) -> (13.1, 3.708846)
  line L11 (10.7, 5.458846) -> (13.1, 5.458846)
  arc A0 (7.95, 8.208846) -> (10.7, 5.458846) centre (10.7, 8.208846) ccw
  line L12 (7.95, 13.158846) -> (7.95, 8.208846)
  line L13 (3.1, 13.158846) -> (7.95, 13.158846)
  line L14 (3.1, 8.258846) -> (3.1, 13.158846)
  arc A1 (1, 6.158846) -> (3.1, 8.258846) centre (1, 8.258846) ccw
  line L15 (0, 6.158846) -> (1, 6.158846)
  line L16 (0, 6.158846) -> (0, 0)
  line L17 (0, 0) -> (2.4, 0)
  line L18 (2.4, 0) -> (2.4, 6.158846)
  line L19 (6.2, 6.158846) -> (2.4, 6.158846)
  line L20 (6.2, 3.117691) -> (6.2, 6.158846)
  line L21 (3.4, 3.117691) -> (6.2, 3.117691)
  line L22 (13.1, 3.708846) -> (24.65, 0.158846)
  point P0 (-16.5, -2.241154)
  constraints: 2 end point
extrude "Vysunutí47" add sketch "Náčrt35" against normal blind 0.8 contours L6 L7 L8 L9 L22
extrude "Vysunutí48" add sketch "Náčrt34" against normal blind 0.8 contours L6 L23 L29 L2 | L29 L23 L16 L9 L2 | L7 L8 L16 L23
sketch "Náčrt17" plane through (-10.5, 0, 0) normal (1, 0, 0) x (0, 0, -1)
  line L0 (-14.182094, 29.090625) -> (-19.645789, 22.579247)
  line L1 (-15.999279, 26.924989) -> (0, 13.5) construction
  line L2 (-22.7, 0) -> (-24.7, 0)
  line L3 (-21.999747, 35.6) -> (-21.999747, 34) construction
  line L4 (-7.193747, 32) -> (-7.193747, 33.5)
  line L5 (-19.645789, 22.579247) -> (-18.594508, 21.697118)
  line L6 (-14.182094, 29.090625) -> (-14.149289, 29.063098)
  line L7 (-23.496813, 29.40051) -> (-17.368457, 24.258209) construction
  line L8 (-17.368457, 24.258209) -> (-15.440095, 26.556343) construction
  line L9 (-15.440095, 26.556343) -> (-21.56845, 31.698644) construction
  line L10 (-21.56845, 31.698644) -> (-20.764966, 32.656199) construction
  arc A0 (-20.764966, 32.656199) -> (-24.300298, 28.442955) centre (-22.532632, 30.549577) ccw construction
  line L11 (-24.300298, 28.442955) -> (-23.496813, 29.40051) construction
  line L12 (-17.75148, 24.579603) -> (-15.823117, 26.877737) construction
  arc A1 (-7.756288, 33.5) -> (-19.6, 15.5) centre (0, 15.5) ccw
  arc A2 (-7.193747, 32) -> (-18, 15.5) centre (0, 15.5) ccw
  line L13 (-24.300298, 28.442955) -> (-30.327049, 33.5) construction
  line L14 (-20.764966, 32.656199) -> (-24.273251, 35.6) construction
  line L15 (-30.327049, 33.5) -> (-30.693747, 33.5) construction
  line L16 (-21.999747, 34) -> (-22.366445, 34) construction
  line L17 (-16.404276, 25.407276) -> (-16.913942, 25.834936)
  point P0 (0, 0)
  point P1 (-19.6, 0)
  point P2 (-14.723569, 25.854541)
  point P3 (-16.787298, 25.72867)
  point P4 (-15.014471, 28.098637)
  dimension "d152" = 40
  dimension "d153" = 14.806
  dimension "d154" = 0.5
  dimension "d155" = 1.6
  dimension "d157" = 8.5
  dimension "d162" = 8
  dimension "d163" = 3
  dimension "d164" = 5.5
  dimension "d165" = 9
  dimension "d166" = 7.5
  dimension "d210" = 23.5
  dimension "d211" = 0.3667
  dimension "d218" = 1.42296
  constraints: 32 end point, 7 perpendicular, 7 point on line, 5 point on circle, 3 horizontal alignment, 3 midpoint, 3 parallel, 2 equal length, 2 horizontal, 2 tangent, 1 centre point, 1 coincident, 1 collinear, 1 vertical
  measures "d152" angle of L2 L1
  measures "d153" distance between parallel lines of L4 L3
  measures "d154" vertical distance of L4.end L3.end
  measures "d155" distance of L3.start L3.end
  measures "d157" distance of L0.start L0.end
  measures "d162" distance between parallel lines of L8 L10
  measures "d163" distance of L7.end L8.end
  measures "d164" distance of L11.start L10.end
  measures "d165" distance from line of L10 point (-14.724, 25.855)
  measures "d166" distance between parallel lines of L12 L10
  measures "d210" distance from line of L4 L15.end
  measures "d211" distance of L3.end L16.end
  measures "d218" distance from line of L17.start L1
extrude "Vysunutí24" add sketch "Náčrt17" against normal blind 8.5
sketch "Náčrt18" plane through (-19, 29.090625, 14.182094) normal (0, 0.6427876, 0.7660444) x (1, 0, 0)
  line L0 (8.5, 0) -> (8.5, -8.5)
  line L1 (8.5, 0) -> (0, 0)
  line L2 (0, -1.294948) -> (0, 0)
  line L3 (0, -8.5) -> (0, -1.294948)
  line L4 (8.5, -8.5) -> (0, -8.5)
  circle A0 centre (4.25, -4.25) radius 4.25
  line L5 (8.5, 0) -> (8.5, -8.5)
  line L6 (8.5, -8.5) -> (0, -8.5)
  point P0 (19, -13.168637)
  point P1 (4.25, -8.5)
  point P2 (0, -4.25)
  point P3 (0, -4.25)
  point P4 (4.25, 0)
  constraints: 3 tangent, 1 centre point
extrude "Vysunutí25" cut sketch "Náčrt18" against normal up to surface contours A0 L3 L2 L1 | L4 L3 A0 round surface about axis through (0, 15.5, 0) along (-1, 0, 0) radius 19.6 far side no
ref_plane "Pracovní rovina2" through (-10.5, 25.72867, 16.787298) normal (0, 0.6427876, 0.7660444) x (1, 0, 0)
sketch "Náčrt19" plane through (-10.5, 25.72867, 16.787298) normal (0, 0.6427876, 0.7660444) x (1, 0, 0)
  arc A0 (-7.304533, 2.955052) -> (-4.25, -4.25) centre (-4.25, 0) ccw
  line L0 (0, -4.25) -> (-4.25, -4.25)
  line L1 (0, 4.25) -> (0, -4.25)
  line L2 (0, 4.25) -> (-4.25, 4.25)
  arc A1 (-4.25, 4.25) -> (-7.304533, 2.955052) centre (-4.25, 0) ccw
  line L3 (-4.25, -3.175426) -> (-7, -1.587713)
  line L4 (-7, -1.587713) -> (-7, 1.587713)
  line L5 (-7, 1.587713) -> (-4.25, 3.175426)
  line L6 (-4.25, 3.175426) -> (-1.5, 1.587713)
  line L7 (-1.5, 1.587713) -> (-1.5, -1.587713)
  line L8 (-1.5, -1.587713) -> (-4.25, -3.175426)
  circle A2 centre (-4.25, 0) radius 1.65
  point P0 (10.5, -8.918637)
  dimension "d167" = 5.5
  dimension "d168" = 3.3
  constraints: 12 end point, 2 coincident, 1 centre point, 1 vertical, 13 other
  measures "d167" distance between parallel lines of L4 L7
  measures "d168" diameter of A2
extrude "Vysunutí26" cut sketch "Náčrt19" along normal through all both and the other way through all contours L3 L4 L5 L6 L7 L8 | A2
extrude "Vysunutí28" add sketch "Náčrt19" along normal blind 2.5 contours A1 L2 L1 L0 A0
sketch "Náčrt20" plane through (-10.5, 27.335639, 18.702409) normal (0, 0.6427876, 0.7660444) x (1, 0, 0)
  arc A0 (-4.25, 4.25) -> (-4.25, -4.25) centre (-4.25, 0) ccw
  line L0 (-4.25, -4.25) -> (0, -4.25)
  line L1 (0, -4.25) -> (0, 4.25)
  line L2 (0, 4.25) -> (-4.25, 4.25)
  line L3 (-4.25, -3.175426) -> (-7, -1.587713)
  line L4 (-7, -1.587713) -> (-7, 1.587713)
  line L5 (-7, 1.587713) -> (-4.25, 3.175426)
  line L6 (-4.25, 3.175426) -> (-1.5, 1.587713)
  line L7 (-1.5, 1.587713) -> (-1.5, -1.587713)
  line L8 (-1.5, -1.587713) -> (-4.25, -3.175426)
  circle A1 centre (-4.25, 0) radius 1.65
  point P0 (10.5, -8.918637)
  dimension "d175" = 3.3
  constraints: 1 centre point, 1 coincident
  measures "d175" diameter of A1
extrude "Vysunutí29" add sketch "Náčrt20" along normal blind 2.4 contours L2 L1 L0 A0 | L3 L4 L5 L6 L7 L8
sketch "Náčrt36" plane through (-8.5, 0, 0) normal (-1, 0, 0) x (0, 0, 1)
  circle A0 centre (45.139, 5) radius 1.7
  line L0 (45.139, 8.889087) -> (49.028087, 5)
  line L1 (41.249913, 5) -> (45.139, 8.889087)
  line L2 (45.139, 1.110913) -> (41.249913, 5)
  line L3 (49.028087, 5) -> (45.139, 1.110913)
  line L4 (41.249913, 5) -> (45.139, 8.889087)
  line L5 (45.139, 8.889087) -> (49.028087, 5)
  line L6 (49.028087, 5) -> (45.139, 1.110913)
  line L7 (45.139, 1.110913) -> (41.249913, 5)
  line L8 (39.639, 9.85) -> (39.639, 0)
  line L9 (39.639, 0) -> (45.582064, 0)
  line L10 (45.582064, 0) -> (46.797798, 0.442491)
  arc A1 (46.797798, 0.442491) -> (45.139, 9.85) centre (45.139, 5) ccw
  line L11 (45.139, 9.85) -> (39.639, 9.85)
  line L12 (33.639, 0) -> (39.639, 0)
  line L13 (39.639, 9.85) -> (39.639, 0)
  line L14 (33.639, 9.85) -> (39.639, 9.85)
  line L15 (33.639, 0) -> (33.639, 9.85)
  line L16 (32.389, 5.860913) -> (45.139, 5.860913)
  line L17 (45.139, 5.860913) -> (45.139, 1.110913)
  line L18 (45.139, 1.110913) -> (32.389, 1.110913)
  line L19 (32.389, 1.110913) -> (32.389, 5.860913)
  line L20 (28.6, 0) -> (33.639, 0)
  line L21 (31.189, 0) -> (31.189, 7.7)
  line L22 (31.189, 7.7) -> (33.589, 7.7)
  line L23 (33.589, 7.7) -> (33.589, 5.860913)
  line L24 (45.139, 2.310913) -> (46.339, 2.310913)
  line L25 (46.339, 2.310913) -> (46.339, 0.275502)
  line L26 (27.2, 7.7) -> (32.5, 7.7)
  line L27 (32.5, 7.7) -> (27.2, 7.7)
  line L28 (27.2, 7.7) -> (29.6, 7.7)
  line L29 (33.7, 7.7) -> (29.6, 7.7)
  line L30 (27.2, 7.7) -> (33.7, 7.7)
  line L31 (33.589, 5.860913) -> (45.139, 2.310913)
  line L32 (33.7, 7.7) -> (39.639, 7.7)
  line L33 (45.139, 1.110913) -> (46.339, 1.110913)
  line L34 (33.7, 7.7) -> (33.7, 5.860913)
  point P0 (0, 0)
  point P1 (33.639, 7.7)
  point P2 (33.639, 5.860913)
  dimension "d299" = 12.75
  dimension "d300" = 4.75
  dimension "d302" = 1.2
  dimension "d303" = 1.2
  dimension "d304" = 1.2
  dimension "d305" = 1.2
  constraints: 26 end point, 11 point on line, 5 perpendicular, 3 parallel, 2 horizontal, 1 vertical
  measures "d299" distance of L16.start L16.end
  measures "d300" distance of L16.end L17.end
  measures "d302" distance between parallel lines of L21 L19
  measures "d303" distance between parallel lines of L19 L23
  measures "d304" distance of L24.start L24.end
  measures "d305" distance between parallel lines of L18 L24
extrude "Vysunutí49" add sketch "Náčrt36" along normal up to surface (12.95 mm away) contours L24 L3 L17 | L33 L25 L10 L9 L8 L18 | L3 L25 L33 | L16 L15 L29 L34 | L8 L12 L15 L18 | L16 L23 L29 L15 | L15 L20 L21 L22 L23 L16 L19 L18
extrude "Vysunutí50" add sketch "Náčrt36" against normal up to next contours L16 L34 L32 L8 | L8 L31 L15 L16 | L8 L18 L15 L31 | L16 L15 L29 L34 | L8 L12 L15 L18 | L31 L16 L15 | L15 L18 L19 L16 L31 | L16 L23 L29 L15 | L15 L20 L21 L22 L23 L16 L19 L18
extrude "Vysunutí51" cut sketch "Náčrt36" along normal blind 3 contours L24 L3 L17 | L3 L25 L33
sketch "Náčrt37" plane through (-21.45, 0.275502, 46.339) normal (-1, 0, 0) x (0, 0, 1)
  line L0 (-12.639, 0.835411) -> (-12.639, -0.275502)
  line L1 (-0.756936, -0.275502) -> (-12.639, -0.275502)
  line L2 (0, 0) -> (-0.756936, -0.275502)
  line L3 (0, 2.035411) -> (0, 0)
  line L4 (-1.2, 2.035411) -> (0, 2.035411)
  line L5 (-1.2, 0.835411) -> (-1.2, 2.035411)
  line L6 (-12.639, 0.835411) -> (-1.2, 0.835411)
  line L7 (-1.2, 2.035411) -> (-12.639, 5.585411)
  line L8 (-13.95, 5.585411) -> (-12.639, 5.585411)
  line L9 (-13.95, 0.835411) -> (-13.95, 5.585411)
  line L10 (-13.95, 0.835411) -> (-1.2, 0.835411)
  point P0 (-46.339, -0.275502)
  constraints: 2 end point
extrude "Vysunutí52" add sketch "Náčrt37" along normal blind 1.2
sketch "Náčrt23" plane through (-10.5, 28.878329, 20.540916) normal (0, 0.6427876, 0.7660444) x (1, 0, 0)
  line L0 (8, 6.236289) -> (8, 5.866304)
  line L1 (8, 6.236289) -> (-4.25, 6.236289)
  line L2 (-4.25, 4.25) -> (-4.25, 6.236289)
  line L3 (-4.25, 4.25) -> (0, 4.25)
  line L4 (0, 5.866304) -> (0, 4.25)
  line L5 (0, 5.866304) -> (8, 5.866304)
  line L6 (0, 5.866304) -> (0, 6.236289)
  line L7 (9.15, 4.779716) -> (9.15, 8.226916)
  line L8 (9.15, 8.226916) -> (8, 8.226916)
  line L9 (8, 5.866304) -> (8, 8.226916)
  line L10 (0, 5.866304) -> (8, 5.866304)
  line L11 (0, 5.866304) -> (0, 4.779716)
  line L12 (9.15, 4.779716) -> (0, 4.779716)
  line L13 (8, 5.866304) -> (8, 4.779716)
  point P0 (10.5, -8.918637)
  point P1 (8, 5.866304)
  point P2 (0, 4.779716)
  constraints: 4 end point, 2 perpendicular, 2 point on line
equation "\"d2\" = d1"
equation "\"d18\" = d17"
